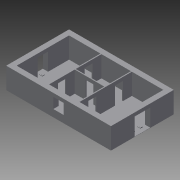
# Autodesk Inventor part: East_Structure_Devices
Saved by Autodesk Inventor 2013 SP2 (Build 170200200, 200)
## iProperties
Created: 2014-07-16
Part Number: East_Structure_Devices
Material: Generic
Document SubType Name: Modeling
Designer: jmw3
Density: 1 g/cm^3
Author: jmw3
Autodesk Inventor part; units mm, degrees
ref_plane "YZ Plane" through (0, 0, 0) normal (1, 0, 0) x (0, 1, 0)
ref_plane "XZ Plane" through (0, 0, 0) normal (0, 1, 0) x (-1, 0, 0)
ref_plane "XY Plane" through (0, 0, 0) normal (0, 0, 1) x (1, 0, 0)
sketch "Sketch1" plane through (0, 0, 0) normal (0, 1, 0) x (-1, 0, 0)
  line L0 (3657.6, -6096) -> (3657.6, 6096)
  line L1 (-3657.6, 6096) -> (-3657.6, -6096)
  line L2 (-5120.64, 0) -> (5120.64, 0) projected
  line L3 (0, -23842.3169) -> (0, 22994.4703) projected
  line L4 (-3048, 1714.5) -> (-3048, -1714.5)
  line L5 (3048, -5486.4) -> (3048, -1828.8)
  line L6 (3048, -1714.5) -> (3048, 1714.5)
  line L7 (3048, 1828.8) -> (3048, 5486.4)
  line L8 (-3048, -1828.8) -> (-3048, -5486.4)
  line L9 (-3048, 5486.4) -> (-3048, 1828.8)
  line L10 (-3048, 1714.5) -> (-3048, -1714.5)
  line L11 (-2009.775, -1828.8) -> (-2009.775, -1714.5)
  line L12 (-1095.375, -1828.8) -> (-1095.375, -1714.5)
  line L13 (-3048, -1714.5) -> (-2009.775, -1714.5)
  line L14 (-1095.375, -1714.5) -> (-57.15, -1714.5)
  line L15 (-3048, -1828.8) -> (-2009.775, -1828.8)
  line L16 (2009.775, -1828.8) -> (2009.775, -1714.5)
  line L17 (1095.375, -1828.8) -> (1095.375, -1714.5)
  line L18 (3048, -1714.5) -> (2009.775, -1714.5)
  line L19 (1095.375, -1714.5) -> (57.15, -1714.5)
  line L20 (3048, -1828.8) -> (2009.775, -1828.8)
  line L21 (1095.375, -1828.8) -> (-1095.375, -1828.8)
  line L22 (-2009.775, -1828.8) -> (-3048, -1828.8)
  line L23 (-1095.375, -1828.8) -> (1095.375, -1828.8)
  line L24 (2009.775, -1828.8) -> (3048, -1828.8)
  line L25 (57.15, -1714.5) -> (1095.375, -1714.5)
  line L26 (2009.775, -1714.5) -> (3048, -1714.5)
  line L27 (-2009.775, 1828.8) -> (-2009.775, 1714.5)
  line L28 (-1095.375, 1828.8) -> (-1095.375, 1714.5)
  line L29 (-3048, 1714.5) -> (-2009.775, 1714.5)
  line L30 (-1095.375, 1714.5) -> (-57.15, 1714.5)
  line L31 (-3048, 1828.8) -> (-2009.775, 1828.8)
  line L32 (3048, 1714.5) -> (2009.775, 1714.5)
  line L33 (3048, 1828.8) -> (2009.775, 1828.8)
  line L34 (2009.775, 1828.8) -> (2009.775, 1714.5)
  line L35 (1095.375, 1828.8) -> (1095.375, 1714.5)
  line L36 (1095.375, 1714.5) -> (57.15, 1714.5)
  line L37 (1095.375, 1828.8) -> (-1095.375, 1828.8)
  line L38 (-2009.775, 1828.8) -> (-3048, 1828.8)
  line L39 (-1095.375, 1828.8) -> (1095.375, 1828.8)
  line L40 (2009.775, 1828.8) -> (3048, 1828.8)
  line L41 (57.15, 1714.5) -> (1095.375, 1714.5)
  line L42 (2009.775, 1714.5) -> (3048, 1714.5)
  line L43 (-57.15, -457.2) -> (57.15, -457.2)
  line L44 (57.15, 457.2) -> (-57.15, 457.2)
  line L45 (-609.6, -6096) -> (-609.6, -5486.4)
  line L46 (609.6, -6096) -> (609.6, -5486.4)
  line L47 (-3048, -5486.4) -> (-609.6, -5486.4)
  line L48 (609.6, -5486.4) -> (3048, -5486.4)
  line L49 (-3657.6, -6096) -> (-609.6, -6096)
  line L50 (609.6, -6096) -> (3657.6, -6096)
  line L51 (914.4, 5486.4) -> (914.4, 6096)
  line L52 (-914.4, 6096) -> (-914.4, 5486.4)
  line L53 (3048, 5486.4) -> (914.4, 5486.4)
  line L54 (-914.4, 5486.4) -> (-3048, 5486.4)
  line L55 (3657.6, 6096) -> (914.4, 6096)
  line L56 (-914.4, 6096) -> (-3657.6, 6096)
  line L57 (-57.15, -1714.5) -> (-57.15, -457.2)
  line L58 (-57.15, 457.2) -> (-57.15, 1714.5)
  line L59 (-57.15, 1714.5) -> (-57.15, 457.2)
  line L60 (-57.15, -457.2) -> (-57.15, -1714.5)
  line L61 (57.15, -1714.5) -> (57.15, -457.2)
  line L62 (57.15, 457.2) -> (57.15, 1714.5)
  line L63 (57.15, 1714.5) -> (57.15, 457.2)
  line L64 (57.15, -457.2) -> (57.15, -1714.5)
  line L65 (-3048, 5486.4) -> (-3048, 1828.8)
  line L66 (-3048, 1828.8) -> (-2009.775, 1828.8)
  line L67 (-2009.775, 1828.8) -> (-2009.775, 1714.5)
  line L68 (-2009.775, 1714.5) -> (-3048, 1714.5)
  line L69 (-3048, 1714.5) -> (-3048, -1714.5)
  line L70 (-3048, -1714.5) -> (-2009.775, -1714.5)
  line L71 (-2009.775, -1714.5) -> (-2009.775, -1828.8)
  line L72 (-2009.775, -1828.8) -> (-3048, -1828.8)
  line L73 (-3048, -1828.8) -> (-3048, -5486.4)
  line L74 (-3048, -5486.4) -> (-609.6, -5486.4)
  line L75 (609.6, -5486.4) -> (3048, -5486.4)
  line L76 (3048, -5486.4) -> (3048, -1828.8)
  line L77 (3048, -1828.8) -> (2009.775, -1828.8)
  line L78 (2009.775, -1828.8) -> (2009.775, -1714.5)
  line L79 (2009.775, -1714.5) -> (3048, -1714.5)
  line L80 (3048, 1714.5) -> (3048, -1714.5)
  line L81 (3048, 1714.5) -> (2009.775, 1714.5)
  line L82 (2009.775, 1714.5) -> (2009.775, 1828.8)
  line L83 (2009.775, 1828.8) -> (3048, 1828.8)
  line L84 (3048, 1828.8) -> (3048, 5486.4)
  point P0 (0, 0)
  point P1 (0, 23842.3169)
  point P2 (0, -22994.4703)
  dimension "d2" = 7315.2
  dimension "d10" = 609.6
  dimension "d13" = 1038.225
  dimension "d14" = 914.4
  dimension "d17" = 114.3
  dimension "d18" = 1038.225
  dimension "d19" = 1038.225
  dimension "d20" = 914.4
  dimension "d21" = 1219.2
  dimension "d23" = 609.6
  dimension "d24" = 4267.2
  dimension "d25" = 1828.8
  dimension "d26" = 12192
  dimension "d27" = 609.6
  dimension "d28" = 114.3
  constraints: 166 end point, 46 perpendicular, 24 collinear, 24 symmetric about line, 23 parallel, 7 horizontal, 8 other
  measures "d2" distance between parallel lines of L0 L1
  measures "d10" distance between parallel lines of L0 L5
  measures "d13" distance between parallel lines of L10 L11
  measures "d14" distance between parallel lines of L11 L12
  measures "d17" distance between parallel lines of L23 L19
  measures "d18" distance of L4.start L29.end
  measures "d19" distance of L6.end L32.end
  measures "d20" distance between parallel lines of L43 L44
  measures "d21" distance between parallel lines of L46 L45
  measures "d23" distance between parallel lines of L49 L47
  measures "d24" distance between parallel lines of L15 L49
  measures "d25" distance between parallel lines of L51 L52
  measures "d26" distance between parallel lines of L50 L55
  measures "d27" distance between parallel lines of L56 L54
  measures "d28" distance between parallel lines of L64 L57
extrude "Extrusion1" add sketch "Sketch1" along normal blind 2438.4
sketch "Sketch2" plane through (-3657.6, 0, -6096) normal (-1, 0, 0) x (0, 0, 1)
  line L0 (0, 0) -> (12192, 0) projected
  line L1 (5486.4, 2032) -> (6705.6, 2032)
  line L2 (6705.6, 2032) -> (6705.6, 812.8)
  line L3 (6705.6, 812.8) -> (5486.4, 812.8)
  line L4 (5486.4, 812.8) -> (5486.4, 2032)
  line L5 (6096, 2926.08) -> (6096, -487.68) projected
  point P0 (6096, 0)
  dimension "d31" = 1219.2
  dimension "d33" = 1219.2
  dimension "d34" = 812.8
  constraints: 8 end point, 2 parallel, 1 horizontal, 1 perpendicular, 1 other
  measures "d31" distance between parallel lines of L2 L4
  measures "d33" distance between parallel lines of L1 L3
  measures "d34" distance between parallel lines of L0 L3
extrude "Extrusion2" cut sketch "Sketch2" against normal up to surface (609.6 mm away)
sketch "Sketch3" plane through (0, 2438.4, 0) normal (0, 1, 0) x (1, 0, 0)
  line L0 (57.15, 1714.5) -> (1095.375, 1714.5) projected
  line L1 (1095.375, 1714.5) -> (1095.375, 1828.8) projected
  line L2 (1095.375, 1828.8) -> (-1095.375, 1828.8) projected
  line L3 (-1095.375, 1828.8) -> (-1095.375, 1714.5) projected
  line L4 (-1095.375, 1714.5) -> (-57.15, 1714.5) projected
  line L5 (-57.15, 1714.5) -> (-57.15, 457.2) projected
  line L6 (-57.15, 457.2) -> (57.15, 457.2) projected
  line L7 (57.15, 457.2) -> (57.15, 1714.5) projected
  line L8 (-57.15, -1714.5) -> (-1095.375, -1714.5) projected
  line L9 (-1095.375, -1714.5) -> (-1095.375, -1828.8) projected
  line L10 (-1095.375, -1828.8) -> (1095.375, -1828.8) projected
  line L11 (1095.375, -1828.8) -> (1095.375, -1714.5) projected
  line L12 (1095.375, -1714.5) -> (57.15, -1714.5) projected
  line L13 (57.15, -1714.5) -> (57.15, -457.2) projected
  line L14 (57.15, -457.2) -> (-57.15, -457.2) projected
  line L15 (-57.15, -457.2) -> (-57.15, -1714.5) projected
  line L16 (3657.6, 6096) -> (609.6, 6096) projected
  line L17 (609.6, 6096) -> (609.6, 5486.4) projected
  line L18 (609.6, 5486.4) -> (3048, 5486.4) projected
  line L19 (3048, 5486.4) -> (3048, 1828.8) projected
  line L20 (3048, 1828.8) -> (2009.775, 1828.8) projected
  line L21 (2009.775, 1828.8) -> (2009.775, 1714.5) projected
  line L22 (2009.775, 1714.5) -> (3048, 1714.5) projected
  line L23 (3048, 1714.5) -> (3048, -1714.5) projected
  line L24 (3048, -1714.5) -> (2009.775, -1714.5) projected
  line L25 (2009.775, -1714.5) -> (2009.775, -1828.8) projected
  line L26 (2009.775, -1828.8) -> (3048, -1828.8) projected
  line L27 (3048, -1828.8) -> (3048, -5486.4) projected
  line L28 (3048, -5486.4) -> (914.4, -5486.4) projected
  line L29 (914.4, -5486.4) -> (914.4, -6096) projected
  line L30 (914.4, -6096) -> (3657.6, -6096) projected
  line L31 (3657.6, -6096) -> (3657.6, 6096) projected
  line L32 (-609.6, 6096) -> (609.6, 6096)
  line L33 (609.6, 6096) -> (609.6, 5486.4)
  line L34 (609.6, 5486.4) -> (-609.6, 5486.4)
  line L35 (-609.6, 5486.4) -> (-609.6, 6096)
  line L36 (-2009.775, 1828.8) -> (-1095.375, 1828.8)
  line L37 (-1095.375, 1828.8) -> (-1095.375, 1714.5)
  line L38 (-1095.375, 1714.5) -> (-2009.775, 1714.5)
  line L39 (-2009.775, 1714.5) -> (-2009.775, 1828.8)
  line L40 (1095.375, 1828.8) -> (2009.775, 1828.8)
  line L41 (2009.775, 1828.8) -> (2009.775, 1714.5)
  line L42 (2009.775, 1714.5) -> (1095.375, 1714.5)
  line L43 (1095.375, 1714.5) -> (1095.375, 1828.8)
  line L44 (-57.15, 457.2) -> (57.15, 457.2)
  line L45 (57.15, 457.2) -> (57.15, -457.2)
  line L46 (57.15, -457.2) -> (-57.15, -457.2)
  line L47 (-57.15, -457.2) -> (-57.15, 457.2)
  line L48 (1095.375, -1714.5) -> (2009.775, -1714.5)
  line L49 (2009.775, -1714.5) -> (2009.775, -1828.8)
  line L50 (2009.775, -1828.8) -> (1095.375, -1828.8)
  line L51 (1095.375, -1828.8) -> (1095.375, -1714.5)
  line L52 (-2009.775, -1714.5) -> (-1095.375, -1714.5)
  line L53 (-1095.375, -1714.5) -> (-1095.375, -1828.8)
  line L54 (-1095.375, -1828.8) -> (-2009.775, -1828.8)
  line L55 (-2009.775, -1828.8) -> (-2009.775, -1714.5)
  line L56 (-914.4, -5486.4) -> (914.4, -5486.4)
  line L57 (914.4, -5486.4) -> (914.4, -6096)
  line L58 (914.4, -6096) -> (-914.4, -6096)
  line L59 (-914.4, -6096) -> (-914.4, -5486.4)
  line L60 (1095.375, 1828.8) -> (2009.775, 1828.8)
  line L61 (2009.775, 1828.8) -> (2009.775, 1714.5)
  line L62 (2009.775, 1714.5) -> (1095.375, 1714.5)
  line L63 (1095.375, 1714.5) -> (1095.375, 1828.8)
  point P0 (0, 0)
  constraints: 64 end point, 16 parallel, 8 horizontal, 8 perpendicular
extrude "Extrusion3" add sketch "Sketch3" against normal blind 406.4 contours L1 L40 L21 L42 | L45 L14 L47 L6 | L3 L38 L39 L36 | L48 L25 L50 L11 | L9 L54 L55 L52 | L34 L35 L32 L17 | L29 L58 L59 L56
sketch "Sketch4" plane through (0, 2032, 0) normal (0, -1, 0) x (1, 0, 0)
  line L0 (914.4, 6096) -> (-914.4, 6096) projected
  line L1 (-914.4, 5486.4) -> (914.4, 5486.4) projected
  line L2 (0, 8534.4) -> (0, -8534.4) projected
  line L3 (-12.7, 6096) -> (12.7, 6096)
  line L4 (12.7, 6096) -> (12.7, 5486.4)
  line L5 (12.7, 5486.4) -> (-12.7, 5486.4)
  line L6 (-12.7, 5486.4) -> (-12.7, 6096)
  point P0 (0, 0)
  dimension "d39" = 25.4
  constraints: 8 end point, 2 parallel, 2 point on line, 1 horizontal, 1 perpendicular, 1 other
  measures "d39" distance between parallel lines of L4 L6
extrude "Extrusion4" add sketch "Sketch4" along normal blind 25.4
sketch "Sketch5" plane through (0, 0, 0) normal (0, -1, 0) x (1, 0, 0)
  line L0 (3657.6, -6096) -> (609.6, -6096) projected
  line L1 (3657.6, 6096) -> (3657.6, -6096) projected
  line L2 (914.4, 6096) -> (3657.6, 6096) projected
  line L3 (914.4, 5486.4) -> (914.4, 6096) projected
  line L4 (3048, 5486.4) -> (914.4, 5486.4) projected
  line L5 (3048, 1828.8) -> (3048, 5486.4) projected
  line L6 (2009.775, 1828.8) -> (3048, 1828.8) projected
  line L7 (2009.775, 1714.5) -> (2009.775, 1828.8) projected
  line L8 (3048, 1714.5) -> (2009.775, 1714.5) projected
  line L9 (3048, -1714.5) -> (3048, 1714.5) projected
  line L10 (2009.775, -1714.5) -> (3048, -1714.5) projected
  line L11 (2009.775, -1828.8) -> (2009.775, -1714.5) projected
  line L12 (3048, -1828.8) -> (2009.775, -1828.8) projected
  line L13 (3048, -5486.4) -> (3048, -1828.8) projected
  line L14 (609.6, -5486.4) -> (3048, -5486.4) projected
  line L15 (609.6, -6096) -> (609.6, -5486.4) projected
  line L16 (-3657.6, 6096) -> (3657.6, 6096)
  line L17 (3657.6, 6096) -> (3657.6, -6096)
  line L18 (3657.6, -6096) -> (-3657.6, -6096)
  line L19 (-3657.6, -6096) -> (-3657.6, 6096)
  point P0 (0, 0)
  constraints: 8 end point, 2 parallel, 1 horizontal, 1 perpendicular
extrude "Extrusion5" add sketch "Sketch5" along normal blind 25.4
sketch "Sketch6" plane through (0, 0, 0) normal (0, 1, 0) x (1, 0, 0)
  circle A0 centre (1549.4, 3657.6) radius 152.4
  line L0 (3048, 5486.4) -> (3048, 1828.8) projected
  line L1 (609.6, 5486.4) -> (3048, 5486.4) projected
  line L2 (1333.5, 3873.5) -> (1765.3, 3873.5)
  line L3 (1765.3, 3873.5) -> (1765.3, 3441.7)
  line L4 (1765.3, 3441.7) -> (1333.5, 3441.7)
  line L5 (1333.5, 3441.7) -> (1333.5, 3873.5)
  circle A1 centre (-1549.4, 3657.6) radius 152.4
  line L6 (-1765.3, 3873.5) -> (-1333.5, 3873.5)
  line L7 (-1333.5, 3873.5) -> (-1333.5, 3441.7)
  line L8 (-1333.5, 3441.7) -> (-1765.3, 3441.7)
  line L9 (-1765.3, 3441.7) -> (-1765.3, 3873.5)
  line L10 (-3048, 5486.4) -> (-609.6, 5486.4) projected
  line L11 (-3048, 1828.8) -> (-3048, 5486.4) projected
  line L12 (57.15, 1714.5) -> (1095.375, 1714.5) projected
  line L13 (2009.775, 1714.5) -> (3048, 1714.5) projected
  line L14 (3048, 1714.5) -> (3048, -1714.5) projected
  circle A2 centre (1549.4, 0) radius 152.4
  line L15 (1333.5, 215.9) -> (1765.3, 215.9)
  line L16 (1765.3, 215.9) -> (1765.3, -215.9)
  line L17 (1765.3, -215.9) -> (1333.5, -215.9)
  line L18 (1333.5, -215.9) -> (1333.5, 215.9)
  line L19 (-1095.375, -1828.8) -> (-1095.375, -1714.5) projected
  line L20 (-2009.775, -1714.5) -> (-2009.775, -1828.8) projected
  line L21 (3048, 1828.8) -> (2009.775, 1828.8) projected
  line L22 (2009.775, 1828.8) -> (2009.775, 1714.5) projected
  line L23 (1095.375, 1828.8) -> (-1095.375, 1828.8) projected
  line L24 (1095.375, 1714.5) -> (1095.375, 1828.8) projected
  circle A3 centre (-1549.4, -3657.6) radius 152.4
  line L25 (-1765.3, -3441.7) -> (-1333.5, -3441.7)
  line L26 (-1333.5, -3441.7) -> (-1333.5, -3873.5)
  line L27 (-1333.5, -3873.5) -> (-1765.3, -3873.5)
  line L28 (-1765.3, -3873.5) -> (-1765.3, -3441.7)
  line L29 (1333.5, -3441.7) -> (1765.3, -3441.7)
  line L30 (1333.5, -3873.5) -> (1333.5, -3441.7)
  circle A4 centre (1549.4, -3657.6) radius 152.4
  line L31 (1765.3, -3441.7) -> (1765.3, -3873.5)
  line L32 (1765.3, -3873.5) -> (1333.5, -3873.5)
  line L33 (3048, -1828.8) -> (3048, -5486.4) projected
  line L34 (3048, -5486.4) -> (914.4, -5486.4) projected
  line L35 (-914.4, -5486.4) -> (-3048, -5486.4) projected
  line L36 (-3048, -5486.4) -> (-3048, -1828.8) projected
  line L37 (-1095.375, -1828.8) -> (1095.375, -1828.8) projected
  line L38 (-3048, -1828.8) -> (-2009.775, -1828.8) projected
  line L39 (609.6, 6096) -> (609.6, 5486.4) projected
  line L40 (-609.6, 5486.4) -> (-609.6, 6096) projected
  line L41 (0, 8534.4) -> (0, -8534.4) projected
  line L42 (-1244.6, 3481.6236) -> (-1549.4, 3305.6473)
  line L43 (-1549.4, 3305.6473) -> (-1854.2, 3481.6236)
  line L44 (-1854.2, 3481.6236) -> (-1854.2, 3833.5764)
  line L45 (-1854.2, 3833.5764) -> (-1549.4, 4009.5527)
  line L46 (-1549.4, 4009.5527) -> (-1244.6, 3833.5764)
  line L47 (-1244.6, 3833.5764) -> (-1244.6, 3481.6236)
  circle A5 centre (0, 5486.4) radius 152.4
  line L48 (215.9, 5702.3) -> (-215.9, 5702.3)
  line L49 (-215.9, 5702.3) -> (-215.9, 5270.5)
  line L50 (-2009.775, -1714.5) -> (-3048, -1714.5) projected
  circle A6 centre (-1549.4, -1714.5) radius 152.4
  line L51 (-1333.5, -1498.6) -> (-1765.3, -1498.6)
  line L52 (-1765.3, -1498.6) -> (-1765.3, -1930.4)
  line L53 (-1333.5, -1498.6) -> (-1765.3, -1930.4)
  line L54 (215.9, 5702.3) -> (-215.9, 5270.5)
  line L55 (914.4, -5486.4) -> (914.4, -6096) projected
  line L56 (-914.4, -6096) -> (-914.4, -5486.4) projected
  circle A7 centre (457.2, -5486.4) radius 152.4
  line L57 (673.1, -5270.5) -> (241.3, -5270.5)
  line L58 (241.3, -5270.5) -> (241.3, -5702.3)
  line L59 (673.1, -5270.5) -> (241.3, -5702.3)
  line L60 (-241.3, -5270.5) -> (-673.1, -5270.5)
  circle A8 centre (-457.2, -5486.4) radius 152.4
  line L61 (-241.3, -5270.5) -> (-673.1, -5702.3)
  line L62 (-673.1, -5270.5) -> (-673.1, -5702.3)
  line L63 (1854.2, -3833.5764) -> (1549.4, -4009.5527)
  line L64 (1549.4, -4009.5527) -> (1244.6, -3833.5764)
  line L65 (1244.6, -3833.5764) -> (1244.6, -3481.6236)
  line L66 (1244.6, -3481.6236) -> (1549.4, -3305.6473)
  line L67 (1549.4, -3305.6473) -> (1854.2, -3481.6236)
  line L68 (1854.2, -3481.6236) -> (1854.2, -3833.5764)
  line L69 (-3048, -1714.5) -> (-3048, 1714.5) projected
  line L70 (2009.775, 1714.5) -> (2009.775, 1828.8) projected
  line L71 (5120.64, 0) -> (-5120.64, 0) projected
  point P0 (0, 0)
  point P1 (1676.4, 3708.4)
  point P2 (1676.4, 3708.4)
  point P3 (-1549.4, 3657.6)
  point P4 (-1244.6, 3657.6)
  point P5 (457.2, -5486.4)
  point P6 (-457.2, -5486.4)
  dimension "d55" = 1498.6
  dimension "d56" = 1828.8
  dimension "d73" = 304.8
  dimension "d84" = 431.8
  dimension "d86" = 215.9
  dimension "d87" = 215.9
  dimension "d91" = 304.8
  dimension "d92" = 431.8
  dimension "d93" = 431.8
  dimension "d94" = 215.9
  dimension "d95" = 215.9
  dimension "d99" = 1828.8
  dimension "d100" = 1498.6
  dimension "d101" = 304.8
  dimension "d102" = 431.8
  dimension "d103" = 431.8
  dimension "d104" = 215.9
  dimension "d105" = 215.9
  dimension "d106" = 1498.6
  dimension "d108" = 304.8
  dimension "d109" = 431.8
  dimension "d110" = 431.8
  dimension "d111" = 215.9
  dimension "d112" = 215.9
  dimension "d113" = 304.8
  dimension "d114" = 431.8
  dimension "d115" = 431.8
  dimension "d116" = 215.9
  dimension "d117" = 215.9
  dimension "d118" = 1498.6
  dimension "d119" = 1828.8
  dimension "d120" = 1498.6
  dimension "d121" = 1828.8
  dimension "d128" = 215.9
  dimension "d136" = 304.8
  dimension "d144" = 304.8
  dimension "d145" = 609.6
  dimension "d146" = 351.9527
  dimension "d147" = 304.8
  dimension "d150" = 431.8
  dimension "d151" = 431.8
  dimension "d152" = 215.9
  dimension "d153" = 431.8
  dimension "d154" = 431.8
  dimension "d155" = 215.9
  dimension "d156" = 304.8
  dimension "d157" = 431.8
  dimension "d158" = 431.8
  dimension "d159" = 215.9
  dimension "d160" = 304.8
  dimension "d161" = 431.8
  dimension "d162" = 431.8
  dimension "d163" = 215.9
  dimension "d164" = 457.2
  dimension "d165" = 457.2
  dimension "d172" = 609.6
  dimension "d175" = 1498.6
  constraints: 88 end point, 12 parallel, 10 coincident, 9 centre point, 9 horizontal, 9 perpendicular, 7 midpoint, 6 point on line, 26 other
  measures "d55" distance from line of L0 A0.centre
  measures "d56" distance from line of L1 A0.centre
  measures "d73" diameter of A0
  measures "d84" distance of L4.end L2.start
  measures "d86" distance from line of A0.centre L3
  measures "d87" distance from line of L2 A0.centre
  measures "d91" diameter of A1
  measures "d92" distance of L7.end L9.start
  measures "d93" distance of L9.start L9.end
  measures "d94" distance from line of A1.centre L7
  measures "d95" distance from line of L6 A1.centre
  measures "d99" distance from line of L10 point (-1549.4, 3657.6)
  measures "d100" distance from line of L11 A1.centre
  measures "d101" diameter of A2
  measures "d102" distance of L15.start L15.end
  measures "d103" distance of L17.end L15.start
  measures "d104" distance from line of A2.centre L18
  measures "d105" distance from line of A2.centre L17
  measures "d106" distance from line of L14 A2.centre
  measures "d108" diameter of A3
  measures "d109" distance of L25.start L25.end
  measures "d110" distance of L28.start L25.start
  measures "d111" distance from line of A3.centre L28
  measures "d112" distance from line of A3.centre L27
  measures "d113" diameter of A4
  measures "d114" distance of L29.start L29.end
  measures "d115" distance of L30.start L29.start
  measures "d116" distance from line of A4.centre L30
  measures "d117" distance from line of A4.centre L32
  measures "d118" distance from line of L33 A4.centre
  measures "d119" distance from line of L34 A4.centre
  measures "d120" distance from line of L36 A3.centre
  measures "d121" distance from line of L35 A3.centre
  measures "d128" distance from line of A0.centre L5
  measures "d136" diameter of A5
  measures "d144" distance of point (-1549.4, 3657.6) point (-1244.6, 3657.6)
  measures "d145" distance between parallel lines of L44 L47
  measures "d146" distance of point (-1549.4, 3657.6) L42.end
  measures "d147" diameter of A6
  measures "d150" distance of L51.start L51.end
  measures "d151" distance of L51.end L52.end
  measures "d152" distance from line of A6.centre L52
  measures "d153" distance of L48.end L49.end
  measures "d154" distance of L48.start L48.end
  measures "d155" distance from line of A5.centre L49
  measures "d156" diameter of A7
  measures "d157" distance of L57.start L57.end
  measures "d158" distance of L57.end L59.end
  measures "d159" distance from line of A7.centre L58
  measures "d160" diameter of A8
  measures "d161" distance of L60.start L60.end
  measures "d162" distance of L60.end L62.end
  measures "d163" distance from line of A8.centre L62
  measures "d164" distance from line of L55 A7.centre
  measures "d165" distance from line of L56 A8.centre
  measures "d172" distance between parallel lines of L65 L68
  measures "d175" distance from line of L69 A6.centre
extrude "Extrusion17" add sketch "Sketch6" along normal blind 76.2 contours A0 | A1 | L71 A2 | A2 L71 | A5 L54 L41 | L41 L54 A5 | L54 A5 L41 | L41 A5 L54 | A3 | A4 | A6 L53 | L53 A6 | A7 L59 | L59 A7 | L61 A8 | A8 L61
extrude "Extrusion18" add sketch "Sketch6" along normal blind 50.8 contours L2 L3 L4 L5 | L6 L7 L8 L9 | L71 L16 L17 L18 A2 | A2 L71 L18 L15 L16 | L54 A5 L41 | L41 A5 L54 | L54 L49 L48 L41 A5 | L41 L48 L54 A5 | L25 L26 L27 L28 | L29 L31 L32 L30 | L53 A6 | A6 L53 L52 L51 | L59 A7 | A7 L59 L58 L57 | L61 A8 L62 L60 | L61 A8 picked at (-82.7306, 5427.6995) picked at (58.7005, 5569.1306) picked at (-1592.4136, -1687.4728) picked at (443.3203, -5425.7518) picked at (-471.0797, -5425.7518)
extrude "Extrusion20" add sketch "Sketch6" along normal blind 25.4 contours L42 L43 L44 L45 L46 L47 | L63 L64 L65 L66 L67 L68
body "Solid1"
